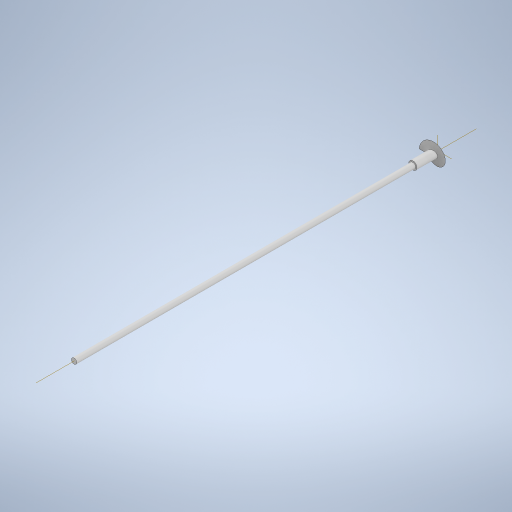
# Autodesk Inventor part: ScrewAnchor
Saved by Autodesk Inventor 2023.2 (Build 272271030, 271C)
## iProperties
Created: 2023-03-03
Part Number: ScrewAnchor
Material: Generisch
Document SubType Name: Modeling
Designer: mehan
Density: 1 g/cm^3
Appearance: Vorgabe
Author: mehan
Autodesk Inventor part; units mm, degrees
ref_plane "YZ Plane" through (0, 0, 0) normal (1, 0, 0) x (0, 1, 0)
ref_plane "XZ Plane" through (0, 0, 0) normal (0, 1, 0) x (-1, 0, 0)
ref_plane "XY Plane" through (0, 0, 0) normal (0, 0, 1) x (1, 0, 0)
sketch "Skizze1" plane through (0, 0, 0) normal (0, 1, 0) x (-1, 0, 0)
  line L0 (0, 0) -> (-9, 0)
  line L1 (-9, 0) -> (-9, 7.6076)
  line L2 (-9, 55) -> (-6, 55)
  line L3 (-6, 55) -> (-6, 800)
  line L4 (-6, 800) -> (0, 800)
  line L5 (0, 800) -> (0, 0)
  line L6 (-9, 7.6076) -> (-9, 55)
  dimension "d0" = 9
  dimension "d1" = 55
  dimension "d3" = 3
  dimension "d4" = 745
  constraints: 14 end point, 5 perpendicular, 2 horizontal
  measures "d0" distance of L0.start L0.end
  measures "d1" distance of L0.end L2.start
  measures "d3" distance of L2.start L2.end
  measures "d4" distance of L2.end L3.end
revolve "Umdrehung1" add sketch "Skizze1" angle 360 about axis through (0, 0, 800) along (0, 0, -1)
sketch "Skizze3" plane through (0, 0, 0) normal (0, 1, 0) x (-1, 0, 0)
  line L0 (25, 1.25) -> (9, 0.45)
  line L1 (25, 1.25) -> (9, 2.05)
  line L2 (9, 55) -> (9, 0) projected
  line L3 (9, 0) -> (9, 3.3582) construction
  line L4 (9, 2.05) -> (9, 0.45)
  point P0 (0, 0)
  constraints: 8 end point, 4 point on line, 1 collinear
coil "Spirale1" sketch "Skizze3" operation add axis through (0, 0, -10) along (0, 0, 1) pitch 15 turns 1 hand right
fillet "Rundung1" radius 7.5 1 edges at (-9, 0, 0)
